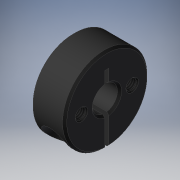
# Autodesk Inventor part: SCSWA6-8b
Saved by Autodesk Inventor 2019 (Build 230136000, 136)
## iProperties
Created: 2024-10-12
Part Number: SCSWA6-8b
Material: Generic
Catalog Web Link: www.cadenas.de
Description: SCSW, PSCSW, SSCSW, SCSWA, SCSWAW-b-Set Collars - Slit 2 Hole/2 Tap - Standard Type - 2 Tap Type
Vendor: MISUMI
Document SubType Name: Modeling
Designer: psAdmin
Manufacturer: MISUMI
Mass: 1.93418 g
Surface Area: 15.2771 cm^2
Volume: 1.93418 cm^3
Density: 1 g/cm^3
Appearance: PSOLRGB-175-175-175
Category: PARTsolutions
Company: MISUMI
Title: SCSWA6-8b
Author: Cadenas PARTsolutions
Comments: Set Collars - Slit 2 Hole/2 Tap - Standard Type - 2 Tap Type
PSOL_IDENT_0: {$CADENAS_DATA/23d-libs/misumi/metric/03_set_collars/scsw_b.prj},199 {VTYP=3D},{NB=SCSWA6-8b},{LINA=
PSOL_IDENT_1: SCSWA6-8b},{NN=SCSW, PSCSW, SSCSW, SCSWA, SCSWAW-b},{DATE=30.11.2021 05:42:06},{GEOMDATE=15.09.2021
PSOL_IDENT_2: 06:01:21},{VERSION=},{LINEID=220},{WBVAR=MAT,ST,BS},{WBNUMERIC=BS}  {NB=SCSWA6-8b},{LINA=SCSWA6-8b},
PSOL_IDENT_3: {KT=DUMMY},{PN=SCSWA6-8},{TYPE=SCSWA},{MAT=2017},{MATA='1045','S45C Equivalent','304','SUS304 Equiva
PSOL_IDENT_4: lent','2017','2017 Aluminum Alloy'},{ST=-},{AC=Hexagon Socket Head Set Screw 1 Pc. (304 Stainless St
PSOL_IDENT_5: eel) },{D=6},{BS=8},{B1=8,10},{D1=20},{M=M3},{THMD=3},{THDMIN=2.459},{ST0='-','-','Clear Anodize','C
PSOL_IDENT_6: lear Anodize'},{DD=3.4},{R=3.00},{W=1.0},{X=6.0},{Y=4.0},{Z=6~6.5},{S=3.5},{P=12},{C=0.5},{L=10},{M1=
PSOL_IDENT_7: M3},{ZZ=6.25},{THMD1=3},{THDMIN1=2.459}
NB: SCSWA6-8b
NN: SCSW, PSCSW, SSCSW, SCSWA, SCSWAW-b
NT: Set Collars - Slit 2 Hole/2 Tap - Standard Type - 2 Tap Type
NBSYN: $PN.b
LINA: SCSWA6-8b
CATALOG: Misumi
PN: SCSWA6-8
MAT: 2017 Aluminum Alloy
ST: -
AC: Hexagon Socket Head Set Screw 1 Pc. (304 Stainless Steel)
D: 6
BS: 8
D1: 20
M: M3
DD: 3.4
R: 3
W: 1
X: 6
Y: 4
Z: 6~6.5
S: 3.5
P: 12
M1: M3
SUPPLIER: MISUMI
ARTICLENO: SCSWA6-8b
BOMINFO: SCSWA6-8b
CREATOR: CADENAS GmbH
Autodesk Inventor part; units mm, degrees
sketch "Sketch_1" plane through (0, 0, 0) normal (0, 0, 1) x (1, 0, 0)
  line L0 (4, 0) -> (-4, 0)
  line L1 (-4, 9.5) -> (-4, 3.5)
  line L2 (-4, 3.5) -> (-3.5, 3)
  line L3 (-3.5, 3) -> (3.5, 3)
  line L4 (3.5, 3) -> (4, 3.5)
  line L5 (4, 3.5) -> (4, 9.5)
  line L6 (4, 9.5) -> (3.5, 10)
  line L7 (3.5, 10) -> (-3.5, 10)
  line L8 (-3.5, 10) -> (-4, 9.5)
  constraints: 18 end point
revolve "Revolution1" add sketch "Sketch_1" angle 360 about axis through (4, 0, 0) along (1, 0, 0)
sketch "Sketch_2" plane through (0, 0, 0) normal (1, 0, 0) x (0, 1, 0)
  line L0 (-10, 0.5) -> (-10, -0.5)
  line L1 (-10, -0.5) -> (6.25, -0.5)
  line L2 (6.25, -0.5) -> (6.25, 0.5)
  line L3 (6.25, 0.5) -> (-10, 0.5)
  constraints: 8 end point
extrude "Extrusion1" cut sketch "Sketch_2" along normal mid plane 8
sketch "Sketch_3" plane through (0, 0, 0) normal (1, 0, 0) x (0, 1, 0)
  line L0 (-6, 10) -> (-6, 0)
  line L1 (-6, 0) -> (-7.7, 0)
  line L2 (-7.7, 0) -> (-7.7, 4)
  line L3 (-7.7, 4) -> (-9, 4)
  line L4 (-9, 4) -> (-9, 10)
  line L5 (-9, 10) -> (-6, 10)
  line L6 (-6, 10) -> (-6, 0)
  constraints: 14 end point
revolve "Revolution2" cut sketch "Sketch_3" angle 360 about axis through (0, -6, 10) along (0, 0, 1)
sketch "Sketch_4" plane through (0, 0, 0) normal (1, 0, 0) x (0, 1, 0)
  line L0 (-6, -9.5) -> (-6, -0.5)
  line L1 (-6, -0.5) -> (-4.5, -0.5)
  line L2 (-4.5, -0.5) -> (-4.7705, -0.7705)
  line L3 (-4.7705, -0.7705) -> (-4.7705, -9.5)
  line L4 (-4.7705, -9.5) -> (-6, -9.5)
  line L5 (-6, -9.5) -> (-6, -0.5)
  constraints: 12 end point
revolve "Revolution3" cut sketch "Sketch_4" angle 360 about axis through (0, -6, -9.5) along (0, 0, -1)
thread "Thread1" size "M3x0.5" class "6H" standard "ISO Metric profile" length 8.1598
sketch "Sketch_7" plane through (0, 0, -6) normal (0, 0, 1) x (1, 0, 0)
  line L0 (4, 0) -> (-4, 0)
  line L1 (-4, 0) -> (-4, 1.5)
  line L2 (-4, 1.5) -> (-3.7295, 1.2295)
  line L3 (-3.7295, 1.2295) -> (3.7295, 1.2295)
  line L4 (3.7295, 1.2295) -> (4, 1.5)
  line L5 (4, 1.5) -> (4, 0)
  line L6 (4, 0) -> (-4, 0)
  constraints: 14 end point
revolve "Revolution4" cut sketch "Sketch_7" angle 360 about axis through (4, 0, -6) along (1, 0, 0)
thread "Thread2" size "M3x0.5" class "6H" standard "ISO Metric profile" full length
sketch "Sketch_8" plane through (0, 0, 6) normal (0, 0, 1) x (1, 0, 0)
  line L0 (4, 0) -> (-4, 0)
  line L1 (-4, 0) -> (-4, 1.5)
  line L2 (-4, 1.5) -> (-3.7295, 1.2295)
  line L3 (-3.7295, 1.2295) -> (3.7295, 1.2295)
  line L4 (3.7295, 1.2295) -> (4, 1.5)
  line L5 (4, 1.5) -> (4, 0)
  line L6 (4, 0) -> (-4, 0)
  constraints: 14 end point
revolve "Revolution5" cut sketch "Sketch_8" angle 360 about axis through (4, 0, 6) along (1, 0, 0)
thread "Thread3" size "M3x0.5" class "6H" standard "ISO Metric profile" full length
ref_plane "body_screw_XY" through (0, -6, 4) normal (0, 0, 1) x (1, 0, 0)
ref_plane "body_screw_YZ" through (0, -6, 4) normal (1, 0, 0) x (0, 1, 0)
ref_plane "body_screw_ZX" through (0, -6, 4) normal (0, 1, 0) x (0, 0, 1)
body "Solid1"
